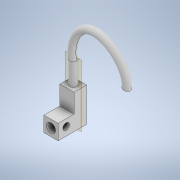
# Autodesk Inventor part: platformHookv1
Saved by Autodesk Inventor 2020 (Build 240168000, 168)
## iProperties
Created: 2019-11-16
Part Number: platformHookv1
Material: Generic
Document SubType Name: Modeling
Designer: xj82b
Density: 1 g/cm^3
Appearance: Default
Author: xj82b
Autodesk Inventor part; units mm, degrees
ref_plane "YZ Plane" through (0, 0, 0) normal (1, 0, 0) x (0, 1, 0)
ref_plane "XZ Plane" through (0, 0, 0) normal (0, 1, 0) x (-1, 0, 0)
ref_plane "XY Plane" through (0, 0, 0) normal (0, 0, 1) x (1, 0, 0)
sketch "Sketch1" plane through (0, 0, 0) normal (0, 0, 1) x (1, 0, 0)
  line L0 (0, 0) -> (7.3125, 0)
  line L1 (7.3125, 0) -> (7.3125, 17.7174)
  line L2 (7.3125, 17.7174) -> (0, 17.7174)
  line L3 (0, 17.7174) -> (0, 0)
  constraints: 8 end point, 2 parallel, 1 horizontal, 1 perpendicular
extrude "Extrusion1" add sketch "Sketch1" along normal blind 6.5
sketch "Sketch2" plane through (0, 17.7174, 0) normal (0, 1, 0) x (1, 0, 0)
  line L0 (7.3125, 0) -> (0, 0) projected
  line L1 (0, 0) -> (0, -6.5) projected
  line L2 (7.3125, -6.5) -> (0, -6.5) projected
  line L3 (7.3125, 0) -> (7.3125, -6.5) projected
  circle A0 centre (3.6562, -3.25) radius 1.8618
  constraints: 1 centre point
extrude "Extrusion2" add sketch "Sketch2" along normal blind 11.5 contours A0
ref_plane "Work Plane1" through (0, 0, 3.25) normal (0, 0, 1) x (1, 0, 0)
sketch "Sketch3" plane through (0, 0, 3.25) normal (0, 0, 1) x (1, 0, 0)
  line L0 (5.5181, 29.2174) -> (1.7944, 29.2174) projected
  spline S0 degree 4 poles (3.6562, 29.2174) (1.2604, 37.8636) (7.2009, 60.1511) (32.7256, 44.0854) (31.2731, 30.1217) knots 0 0 0 0 0 1 1 1 1 1
  point P0 (0, 0)
  point P1 (4.4619, 39.176)
  point P2 (11.5543, 46.3185)
  point P3 (23.5265, 44.0553)
  constraints: 1 midpoint, 5 other
sketch "Sketch4" plane through (3.6562, 29.2174, 3.25) normal (0, 1, 0) x (1, 0, 0)
  circle A0 centre (0, 0) radius 1.8618 projected
  point P0 (-3.6562, 3.25)
sweep "Sweep1" add profiles "Sketch4" path "Sketch3" path curves S0
sketch "Sketch5" plane through (0, 0, 6.5) normal (0, 0, 1) x (1, 0, 0)
  line L0 (0, 17.7174) -> (0, 0) projected
  line L1 (7.3125, 0) -> (7.3125, 17.7174) projected
  line L2 (0, 0) -> (7.3125, 0)
  line L3 (7.3125, 0) -> (7.3125, 7.8965)
  line L4 (7.3125, 7.8965) -> (0, 7.8965)
  line L5 (0, 7.8965) -> (0, 0)
  constraints: 8 end point, 2 parallel, 1 horizontal, 1 perpendicular, 1 point on line
extrude "Extrusion3" add sketch "Sketch5" along normal blind 8.25
sketch "Sketch6" plane through (0, 0, 14.75) normal (0, 0, 1) x (1, 0, 0)
  circle A0 centre (3.6562, 3.9482) radius 2.358
  line L0 (7.3125, 7.8965) -> (0, 7.8965) projected
  line L1 (0, 7.8965) -> (0, 0) projected
  line L2 (0, 0) -> (7.3125, 0) projected
  line L3 (7.3125, 0) -> (7.3125, 7.8965) projected
  point P0 (7.3125, 3.9482)
  point P1 (3.6562, 0)
  constraints: 2 midpoint, 1 centre point, 1 horizontal alignment, 1 vertical alignment
extrude "Extrusion4" cut sketch "Sketch6" against normal through all contours A0
sketch "Sketch7" plane through (7.3125, 0, 0) normal (1, 0, 0) x (0, 0, -1)
  line L0 (0, 0) -> (0, 17.7174) projected
  line L1 (0, 17.7174) -> (-6.5, 17.7174) projected
  line L2 (-6.5, 7.8965) -> (-6.5, 17.7174) projected
  line L3 (-6.5, 7.8965) -> (-14.75, 7.8965) projected
  line L4 (-14.75, 0) -> (-14.75, 7.8965) projected
  line L5 (0, 0) -> (-14.75, 0) projected
  circle A0 centre (-10.625, 4.3798) radius 1.7093
  constraints: 1 centre point
extrude "Extrusion5" cut sketch "Sketch7" against normal up to next contours A0
body "Solid1"
